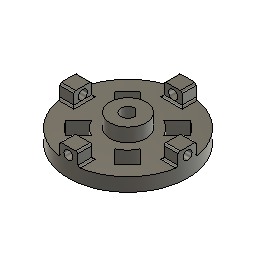
Cuplinug (Autodesk Fusion 360 design; units mm, degrees)
part number: 2025-04-25-17-17-15-757
Autodesk Fusion 360 part; units mm, degrees
note: some values were not read from the file. Set by a fixed rule: which sketch regions a step uses.
sketch "Sketch1" plane through (0, 0, 0) normal (0, 1, 0) x (1, 0, 0)
  line L0 (0.2505, 3.9921) -> (3.9921, 0.2505)
  arc A0 (0.2505, 3.9921) -> (3.9921, 0.2505) centre (0, 0) ccw
  circle A1 centre (0, 0) radius 33.1
  dimension "d1" = 8
  dimension "d2" = 3
  dimension "d3" = 66.2
  constraint coincident A0.centre A1.centre
  constraint concentric A0 A1
  measures "d1" diameter of A0
  measures "d2" distance of A0.centre L0
  measures "d3" diameter of A1
extrude "Extrude1" add sketch "Sketch1" along normal blind 7.5
sketch "Sketch2" plane through (0, 7.5, 0) normal (0, 1, 0) x (-1, 0, 0)
  arc A0 (-0.2505, -3.9921) -> (-3.9921, -0.2505) centre (0, 0) ccw
  line L0 (-0.2505, -3.9921) -> (-3.9921, -0.2505)
  circle A1 centre (0, 0) radius 33.1
  circle A2 centre (0, 0) radius 10
  line L1 (32.7202, -5) -> (25, -5)
  line L2 (25, -5) -> (25, 5)
  line L3 (25, 5) -> (32.7202, 5)
  line L4 (32.9668, -2.9668) -> (25, 5) construction
  line L5 (25, -5) -> (32.9668, 2.9668) construction
  line L6 (5, 32.7202) -> (5, 25)
  line L7 (5, 25) -> (-5, 25)
  line L8 (-5, 25) -> (-5, 32.7202)
  line L9 (-32.7202, 5) -> (-25, 5)
  line L10 (-25, 5) -> (-25, -5)
  line L11 (-25, -5) -> (-32.7202, -5)
  line L12 (-5, -32.7202) -> (-5, -25)
  line L13 (-5, -25) -> (5, -25)
  line L14 (5, -25) -> (5, -32.7202)
  point P0 (30, 0)
  dimension "d6" = 20
  dimension "d10" = 360
  constraint coincident A0.centre A1.centre
  constraint horizontal L1
  constraint perpendicular L1 L2
  constraint parallel L1 L3
  constraint coincident L4 P0
  constraint coincident L5 P0
  constraint coincident A1 L1.start
  constraint coincident A1 L3.end
  constraint coincident A1 L4.start
  constraint coincident A1 L5.end
  measures "d6" diameter of A2
extrude "Extrude2" add sketch "Sketch2" along normal blind 7.5 contours A1 L1 L2 L3 | A1 L6 L7 L8 | A1 L12 L13 L14 | A1 L9 L10 L11 | A2
ref_plane "WorkPlane1" through (0, 12.125, 0) normal (0.707107, 0, -0.707107) x (0, 1, 0)
sketch "Sketch3" plane through (0, 0, 0) normal (0.707107, 0, -0.707107) x (0, 1, 0)
  circle A0 centre (11.5, 0) radius 1.5
  line L0 (15, -10) -> (15, 10)
  dimension "d12" = 3
  dimension "d13" = 3.5
  measures "d12" diameter of A0
  measures "d13" distance of A0.centre L0
extrude "Extrude3" cut sketch "Sketch3" along normal blind 20
ref_plane "WorkPlane2" through (33.1, 7.3335, 0) normal (1, 0, 0) x (0, 0, 1)
sketch "Sketch4" plane through (33.1, 0, 0) normal (1, 0, 0) x (0, 0, -1)
  circle A0 centre (0, 11) radius 2.5
  line L0 (5, 15) -> (-5, 15)
  dimension "d17" = 5
  dimension "d18" = 4
  measures "d17" diameter of A0
  measures "d18" distance of A0.centre L0
extrude "Extrude4" cut sketch "Sketch4" against normal blind 11
pattern_circular "C-Pattern1" count 4 over 360 about axis through (0, 1.75, 0) along (0, 1, 0) of "Extrude4"
fillet "Fillet1" radius 1 20 edges at (5, 7.5, 28.8601) (5, 15, 28.8601) (-5, 15, 28.8601) (-28.8601, 15, 5) (-28.8601, 7.5, 5) (-28.8601, 15, -5) (-5, 15, -28.8601) (5, 15, -28.8601) (5, 7.5, -28.8601) (28.8601, 15, -5) (28.8601, 15, 5) (28.8601, 7.5, 5) (28.8601, 7.5, -5) (-5, 7.5, 28.8601) (-5, 7.5, -28.8601) (-28.8601, 7.5, -5) (25, 7.5, 0) (0, 7.5, 25) (-25, 7.5, 0) (0, 7.5, -25)
sketch "Sketch5" plane through (0, 7.5, 0) normal (0, 1, 0) x (-1, 0, 0)
  line L0 (-32.5517, 6) -> (-24, 6)
  line L1 (-24, 6) -> (-24, -6)
  line L2 (-24, -6) -> (-32.5517, -6)
  arc A0 (-32.5517, -6) -> (-6, -32.5517) centre (0, 0) ccw
  line L3 (-6, -32.5517) -> (-6, -24)
  line L4 (-6, -24) -> (6, -24)
  line L5 (6, -24) -> (6, -32.5517)
  arc A1 (6, -32.5517) -> (32.5517, -6) centre (0, 0) ccw
  line L6 (32.5517, -6) -> (24, -6)
  line L7 (24, -6) -> (24, 6)
  line L8 (24, 6) -> (32.5517, 6)
  arc A2 (32.5517, 6) -> (6, 32.5517) centre (0, 0) ccw
  line L9 (6, 32.5517) -> (6, 24)
  line L10 (6, 24) -> (-6, 24)
  line L11 (-6, 24) -> (-6, 32.5517)
  arc A3 (-6, 32.5517) -> (-32.5517, 6) centre (0, 0) ccw
  circle A4 centre (0, 0) radius 10
  circle A5 centre (0.128, 0.128) radius 15
  circle A6 centre (0, 0) radius 25
  line L12 (-30.4056, -23.3345) -> (23.5906, 30.6617)
  line L13 (23.5906, 30.6617) -> (30.6617, 23.5906)
  line L14 (30.6617, 23.5906) -> (-23.3345, -30.4056)
  line L15 (-23.3345, -30.4056) -> (-30.4056, -23.3345)
  line L16 (-30.4056, -23.3345) -> (30.6617, 23.5906) construction
  line L17 (23.5906, 30.6617) -> (-23.3345, -30.4056) construction
  line L18 (30.6617, 23.5906) -> (-23.3345, -30.4056)
  line L19 (23.5906, 30.6617) -> (-23.3345, -30.4056) construction
  line L20 (-30.4056, -23.3345) -> (30.6617, 23.5906) construction
  line L21 (-30.4056, -23.3345) -> (23.5906, 30.6617)
  line L22 (-23.3345, -30.4056) -> (-30.4056, -23.3345)
  line L23 (23.5906, 30.6617) -> (30.6617, 23.5906)
  line L24 (-23.3345, 30.6617) -> (30.6617, -23.3345)
  line L25 (23.5906, -30.4056) -> (-30.4056, 23.5906)
  line L26 (-30.4056, 23.5906) -> (30.6617, -23.3345) construction
  line L27 (-30.4056, 23.5906) -> (30.6617, -23.3345) construction
  line L28 (23.5906, -30.4056) -> (-23.3345, 30.6617) construction
  line L29 (30.6617, -23.3345) -> (23.5906, -30.4056)
  line L30 (-30.4056, 23.5906) -> (-23.3345, 30.6617)
  point P0 (0.128, 0.128)
  point P1 (0.128, 0.128)
  dimension "d25" = 30
  constraint coincident A0.centre A1.centre
  constraint perpendicular L12 L13
  constraint parallel L12 L14
  constraint parallel L13 L15
  constraint coincident L16 P1
  constraint coincident L17 P1
  constraint coincident P1 P0
  constraint perpendicular L21 L23
  constraint parallel L18 L21
  constraint parallel L22 L23
  constraint parallel L24 L25
  constraint coincident P1 L28
  constraint coincident P1 L27
  measures "d25" diameter of A5
extrude "Extrude5" cut sketch "Sketch5" against normal blind 18 contours A5 A6 L24 L25 | A5 A6 L12 L14 L18 L21 | A5 A6 L12 L14 L18 L21 | A5 A6 L24 L25
equation "d11 = 45 deg + 45 deg + 45 deg"
